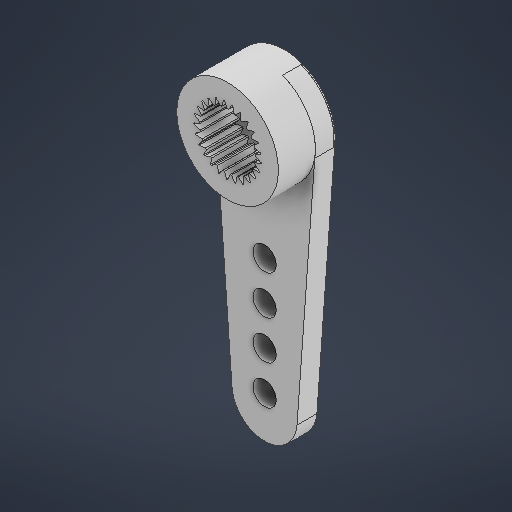
# Autodesk Inventor part: servoarm
Saved by Autodesk Inventor 2026.1 (Build 301233000, 233)
## iProperties
Created: 2026-01-25
Part Number: servoarm
Material: Generic
Document SubType Name: Modeling
Designer: mateo
Density: 1 g/cm^3
Appearance: Default
Author: mateo
Autodesk Inventor part; units mm, degrees
ref_plane "YZ Plane" through (0, 0, 0) normal (1, 0, 0) x (0, 1, 0)
ref_plane "XZ Plane" through (0, 0, 0) normal (0, 1, 0) x (-1, 0, 0)
ref_plane "XY Plane" through (0, 0, 0) normal (0, 0, 1) x (1, 0, 0)
sketch "Sketch2" plane through (176.6929, 204.3818, 5.2281) normal (0, 0, 1) x (1, 0, 0)
  circle A0 centre (2.9232, 3.4092) radius 1.1834 projected
  circle A1 centre (2.9144, 3.4084) radius 4.4788 projected
  circle A2 centre (2.9144, 3.4084) radius 4.4788
  circle A3 centre (2.9144, 3.4084) radius 2.45
  point P0 (-176.6929, -204.3818)
  dimension "d1" = 4.9
  constraints: 2 centre point, 2 coincident, 1 concentric
  measures "d1" diameter of A3
extrude "Extrusion1" add sketch "Sketch2" against normal blind 5 contours A1
sketch "Sketch3" plane through (176.7667, 185.9223, 1.9791) normal (0, 0, 1) x (1, 0, 0)
  circle A0 centre (2.8406, 21.8679) radius 4.4788 projected
  circle A1 centre (2.8455, 0.2215) radius 2.8689 projected
  line L0 (-1.6382, 21.8679) -> (-0.0155, 0.0091)
  line L1 (7.3194, 21.8679) -> (5.7066, 0.0104)
  circle A2 centre (2.8519, 11.3117) radius 1.0301 projected
  circle A3 centre (2.8526, 7.8787) radius 1.0313 projected
  circle A4 centre (2.8531, 4.4493) radius 1.0279 projected
  circle A5 centre (2.8511, 1.0153) radius 1.0308 projected
  circle A6 centre (2.8519, 11.3117) radius 1.0301
  circle A7 centre (2.8526, 7.8787) radius 1.0313
  circle A8 centre (2.8531, 4.4493) radius 1.0279
  circle A9 centre (2.8511, 1.0153) radius 1.0308
  arc A10 (-0.0155, 0.0091) -> (5.7066, 0.0104) centre (2.8455, 0.2215) ccw
  point P0 (-176.7667, -185.9223)
  point P1 (7.2709, 21.2105)
  point P2 (-1.5891, 21.2066)
  constraints: 6 point on circle, 5 centre point, 5 coincident, 5 concentric, 4 end point, 2 tangent
extrude "Extrusion2" add sketch "Sketch3" against normal up to surface (1.751 mm away) contours L1 A1 L0 A0 | A1
sketch "Sketch4" plane through (182.4359, 208.0709, 0.3432) normal (0, 0, -1) x (-1, 0, 0)
  circle A0 centre (2.8144, -0.2785) radius 1.182 projected
  circle A1 centre (2.8144, -0.2785) radius 4.4717
  point P0 (182.4359, -208.0709)
  constraints: 1 centre point, 1 coincident
extrude "Extrusion3" add sketch "Sketch4" against normal up to surface (1.6359 mm away)
sketch "Sketch5" plane through (179.6073, 207.7901, 5.2281) normal (0, 0, 1) x (1, 0, 0)
  circle A0 centre (0, 0) radius 2.45 projected
  line L0 (1.7345, 1.7303) -> (2.29, 1.8759)
  line L1 (2.29, 1.8759) -> (2.3396, 1.8165)
  line L2 (2.3396, 1.8165) -> (2.0463, 1.3472)
  line L3 (1.2497, 2.1073) -> (1.7515, 2.3864)
  line L4 (1.8143, 2.3413) -> (1.647, 1.8138)
  line L5 (1.7515, 2.3864) -> (1.8143, 2.3413)
  line L6 (0.6864, 2.3519) -> (1.103, 2.7471)
  line L7 (1.1751, 2.7189) -> (1.1442, 2.1664)
  line L8 (1.103, 2.7471) -> (1.1751, 2.7189)
  line L9 (0.0799, 2.4487) -> (0.3852, 2.9351)
  line L10 (0.462, 2.9257) -> (0.5695, 2.3829)
  line L11 (0.3852, 2.9351) -> (0.462, 2.9257)
  line L12 (-0.5316, 2.3916) -> (-0.3568, 2.9386)
  line L13 (-0.2801, 2.9487) -> (-0.041, 2.4497)
  line L14 (-0.3568, 2.9386) -> (-0.2801, 2.9487)
  line L15 (-1.1097, 2.1843) -> (-1.0764, 2.7576)
  line L16 (-1.0046, 2.7864) -> (-0.6489, 2.3625)
  line L17 (-1.0764, 2.7576) -> (-1.0046, 2.7864)
  line L18 (-1.618, 1.8397) -> (-1.7284, 2.4032)
  line L19 (-1.666, 2.449) -> (-1.2161, 2.1269)
  line L20 (-1.7284, 2.4032) -> (-1.666, 2.449)
  line L21 (-2.0247, 1.3795) -> (-2.2718, 1.8979)
  line L22 (-2.2227, 1.9578) -> (-1.7068, 1.7577)
  line L23 (-2.2718, 1.8979) -> (-2.2227, 1.9578)
  line L24 (-2.3042, 0.8327) -> (-2.6724, 1.2733)
  line L25 (-2.6398, 1.3435) -> (-2.0903, 1.278)
  line L26 (-2.6724, 1.2733) -> (-2.6398, 1.3435)
  line L27 (-2.4388, 0.2335) -> (-2.9051, 0.5687)
  line L28 (-2.891, 0.6448) -> (-2.3424, 0.718)
  line L29 (-2.9051, 0.5687) -> (-2.891, 0.6448)
  line L30 (-2.4203, -0.3804) -> (-2.9552, -0.1716)
  line L31 (-2.9605, -0.0944) -> (-2.4474, 0.1129)
  line L32 (-2.9552, -0.1716) -> (-2.9605, -0.0944)
  line L33 (-2.2497, -0.9703) -> (-2.8197, -0.9012)
  line L34 (-2.844, -0.8277) -> (-2.3986, -0.4993)
  line L35 (-2.8197, -0.9012) -> (-2.844, -0.8277)
  line L36 (-1.9377, -1.4993) -> (-2.507, -1.5741)
  line L37 (-2.5488, -1.509) -> (-2.1991, -1.0801)
  line L38 (-2.507, -1.5741) -> (-2.5488, -1.509)
  line L39 (-1.5039, -1.9341) -> (-2.0368, -2.1481)
  line L40 (-2.0935, -2.0954) -> (-1.8614, -1.5931)
  line L41 (-2.0368, -2.1481) -> (-2.0935, -2.0954)
  line L42 (-0.9757, -2.2473) -> (-1.4386, -2.5872)
  line L43 (-1.5066, -2.5502) -> (-1.4067, -2.0059)
  line L44 (-1.4386, -2.5872) -> (-1.5066, -2.5502)
  line L45 (-0.3862, -2.4194) -> (-0.75, -2.8636)
  line L46 (-0.825, -2.8448) -> (-0.8637, -2.2927)
  line L47 (-0.75, -2.8636) -> (-0.825, -2.8448)
  line L48 (0.2276, -2.4394) -> (-0.0143, -2.9602)
  line L49 (-0.0917, -2.9606) -> (-0.2663, -2.4355)
  line L50 (-0.0143, -2.9602) -> (-0.0917, -2.9606)
  line L51 (0.8271, -2.3062) -> (0.7223, -2.8707)
  line L52 (0.6475, -2.8904) -> (0.3477, -2.4252)
  line L53 (0.7223, -2.8707) -> (0.6475, -2.8904)
  line L54 (1.3747, -2.028) -> (1.4136, -2.6009)
  line L55 (1.3459, -2.6385) -> (0.9399, -2.2625)
  line L56 (1.4136, -2.6009) -> (1.3459, -2.6385)
  line L57 (1.8358, -1.6224) -> (2.016, -2.1677)
  line L58 (1.9598, -2.2209) -> (1.473, -1.9577)
  line L59 (2.016, -2.1677) -> (1.9598, -2.2209)
  line L60 (2.1816, -1.1149) -> (2.4917, -1.5982)
  line L61 (2.4506, -1.6637) -> (1.9136, -1.5299)
  line L62 (2.4917, -1.5982) -> (2.4506, -1.6637)
  line L63 (2.3904, -0.5373) -> (2.8109, -0.9283)
  line L64 (2.7873, -1.002) -> (2.234, -1.0059)
  line L65 (2.8109, -0.9283) -> (2.7873, -1.002)
  line L66 (2.4489, 0.074) -> (2.9534, -0.2001)
  line L67 (2.949, -0.2774) -> (2.414, -0.4187)
  line L68 (2.9534, -0.2001) -> (2.949, -0.2774)
  line L69 (2.3535, 0.6807) -> (2.9104, 0.5407)
  line L70 (2.9253, 0.4647) -> (2.4422, 0.1947)
  line L71 (2.9104, 0.5407) -> (2.9253, 0.4647)
  line L72 (2.1103, 1.2446) -> (2.6845, 1.2475)
  line L73 (2.7178, 1.1776) -> (2.3171, 0.796)
  line L74 (2.6845, 1.2475) -> (2.7178, 1.1776)
  point P0 (-179.6073, -207.7901)
  point P1 (2.1816, -1.1149)
  point P2 (1.9136, -1.5299)
  point P3 (1.8358, -1.6224)
  point P4 (1.473, -1.9577)
  point P5 (1.3747, -2.028)
  point P6 (0.9399, -2.2625)
  point P7 (0.8271, -2.3062)
  point P8 (0.3477, -2.4252)
  point P9 (0.2276, -2.4394)
  point P10 (-0.2663, -2.4355)
  point P11 (-0.3862, -2.4194)
  point P12 (-0.8637, -2.2927)
  point P13 (2.3904, -0.5373)
  point P14 (2.234, -1.0059)
  point P15 (2.4489, 0.074)
  point P16 (2.414, -0.4187)
  point P17 (-0.9757, -2.2473)
  point P18 (-1.4067, -2.0059)
  point P19 (-1.5039, -1.9341)
  point P20 (-1.8614, -1.5931)
  point P21 (-1.9377, -1.4993)
  point P22 (-2.1991, -1.0801)
  point P23 (-2.2497, -0.9703)
  point P24 (-2.3986, -0.4993)
  point P25 (-2.4203, -0.3804)
  point P26 (-2.4474, 0.1129)
  point P27 (-2.4388, 0.2335)
  point P28 (-2.3424, 0.718)
  point P29 (-2.3042, 0.8327)
  point P30 (-2.0903, 1.278)
  point P31 (-2.0247, 1.3795)
  point P32 (-1.7068, 1.7577)
  point P33 (-1.618, 1.8397)
  point P34 (-1.2161, 2.1269)
  point P35 (2.3535, 0.6807)
  point P36 (2.4422, 0.1947)
  point P37 (2.1103, 1.2446)
  point P38 (2.3171, 0.796)
  point P39 (1.2497, 2.1073)
  point P40 (1.647, 1.8138)
  point P41 (-1.1097, 2.1843)
  point P42 (-0.6489, 2.3625)
  point P43 (0.6864, 2.3519)
  point P44 (1.1442, 2.1664)
  point P45 (0.0799, 2.4487)
  point P46 (0.5695, 2.3829)
  point P47 (-0.5316, 2.3916)
  point P48 (-0.041, 2.4497)
  dimension "d10" = 360
  constraints: 150 end point, 179 other
extrude "Extrusion4" cut sketch "Sketch5" against normal up to surface (3.249 mm away) contours A0 L66 L68 L67 | A0 L69 L71 L70 | L63 L65 L64 A0 | A0 L72 L74 L73 | L60 L62 L61 A0 | A0 L0 L1 L2 | L57 L59 L58 A0 | A0 L3 L5 L4 | L54 L56 L55 A0 | A0 L6 L8 L7 | L51 L53 L52 A0 | A0 L9 L11 L10 | L48 L50 L49 A0 | A0 L12 L14 L13 | L45 L47 L46 A0 | A0 L15 L17 L16 | L42 L44 L43 A0 | A0 L18 L20 L19 | L39 L41 L40 A0 | A0 L21 L23 L22 | L36 L38 L37 A0 | A0 L24 L26 L25 | L33 L35 L34 A0 | A0 L27 L29 L28 | L30 L32 L31 A0
body "Solid1"
